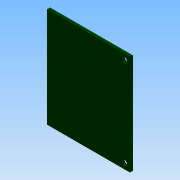
# Autodesk Inventor part: board
Saved by Autodesk Inventor 2015 (Build 190159000, 159)
## iProperties
Created: 2015-06-10
Part Number: board
Material: Générique
Document SubType Name: Modeling
Designer: Gregwar
Density: 1 g/cm^3
Appearance: Par défaut
Author: Gregwar
Autodesk Inventor part; units mm, degrees
ref_plane "YZ Plane" through (0, 0, 0) normal (1, 0, 0) x (0, 1, 0)
ref_plane "XZ Plane" through (0, 0, 0) normal (0, 1, 0) x (-1, 0, 0)
ref_plane "XY Plane" through (0, 0, 0) normal (0, 0, 1) x (1, 0, 0)
sketch "Esquisse1" plane through (0, 0, 0) normal (0, 1, 0) x (-1, 0, 0)
  line L0 (0, 0) -> (45.5, 0)
  line L1 (45.5, 0) -> (45.5, -55)
  line L2 (45.5, -55) -> (0, -55)
  line L3 (0, -55) -> (0, 0)
  line L4 (3, 0) -> (3, -55) construction
  circle A0 centre (3, -3) radius 1.5
  line L5 (45.5, -27.5) -> (0, -27.5) construction
  circle A1 centre (3, -52) radius 1.5
  dimension "d0" = 3
  dimension "d1" = 45.5
  dimension "d2" = 55
  dimension "d3" = 49
  dimension "d4" = 3
  constraints: 12 end point, 3 point on line, 2 centre point, 2 midpoint, 2 parallel, 1 horizontal, 1 perpendicular, 1 symmetric about line, 1 vertical, 1 other
  measures "d0" diameter of A1
  measures "d1" distance between parallel lines of L1 L3
  measures "d2" distance between parallel lines of L0 L2
  measures "d3" distance of A0.centre A1.centre
  measures "d4" distance from line of L3 A0.centre
extrude "Extrusion1" add sketch "Esquisse1" along normal blind 1.6
